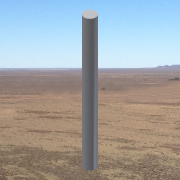
# Autodesk Inventor part: feed-spacer
Saved by Autodesk Inventor 2013 SP2 (Build 170200200, 200)
## iProperties
Company: HERA Project
Created: 2013-06-03
Part Number: feed-spacer
Material: Acetal Resin, White
Document SubType Name: Modeling
Designer: Rich Bradley
Density: 1.425 g/cm^3
Description: Feed disk spacer
Mass: 26.3641 g
Surface Area: 60.8049 cm^2
Volume: 18.5012 cm^3
Author: David DeBoer
Title: Feed spacer
Autodesk Inventor part; units mm, degrees
ref_plane "YZ Plane" through (0, 0, 0) normal (1, 0, 0) x (0, 1, 0)
ref_plane "XZ Plane" through (0, 0, 0) normal (0, 1, 0) x (-1, 0, 0)
ref_plane "XY Plane" through (0, 0, 0) normal (0, 0, 1) x (1, 0, 0)
sketch "Sketch1" plane through (0, 0, 0) normal (0, 1, 0) x (-1, 0, 0)
  circle A0 centre (0, 0) radius 6.35
  dimension "d0" = 12.7
  constraints: 1 centre point, 1 coincident
  measures "d0" diameter of A0
extrude "Extrusion1" add sketch "Sketch1" along normal blind 146.05
body "Solid1"
